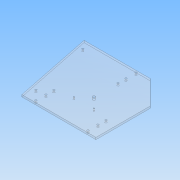
# Autodesk Inventor part: Top_Separator Backboard 2 Lanes
Saved by Autodesk Inventor 2018.1 (Build 221171000, 171)
## iProperties
Created: 2019-03-20
Part Number: Top_Separator Backboard 2 Lanes
Material: PMMA Plastic
Document SubType Name: Modeling
Designer: James
Density: 1.188 g/cm^3
Appearance: Polycarbonate - Clear
Author: James
Autodesk Inventor part; units mm, degrees
ref_plane "YZ Plane" through (0, 0, 0) normal (1, 0, 0) x (0, 1, 0)
ref_plane "XZ Plane" through (0, 0, 0) normal (0, 1, 0) x (-1, 0, 0)
ref_plane "XY Plane" through (0, 0, 0) normal (0, 0, 1) x (1, 0, 0)
sketch "Sketch1" plane through (0, 0, 0) normal (0, 0, 1) x (1, 0, 0)
  line L0 (0, 0) -> (-39.6732, 195)
  line L1 (-39.6732, 195) -> (185, 195)
  line L2 (185, 195) -> (185, 0)
  line L3 (185, 0) -> (0, 0)
  dimension "d0" = 195
  dimension "d1" = 78.5
  dimension "d2" = 185
  constraints: 8 end point, 2 perpendicular, 1 horizontal
  measures "d0" distance of L1.end L2.end
  measures "d1" angle of L3 L0
  measures "d2" distance of L2.end L0.start
extrude "Extrusion1" add sketch "Sketch1" along normal blind 5
sketch "Sketch2" plane through (0, 0, 5) normal (0, 0, 1) x (1, 0, 0)
  line L0 (0, 0) -> (185, 0) projected
  point P0 (95, 165)
  point P1 (95, 145)
  point P2 (30, 50)
  point P3 (30, 30)
  point P4 (160, 50)
  point P5 (160, 30)
  point P6 (95, 190)
  point P7 (30, 5)
  point P8 (160, 5)
  dimension "d5" = 20
  dimension "d7" = 20
  dimension "d15" = 25
  dimension "d16" = 95
  dimension "d20" = 5
  dimension "d21" = 30
  dimension "d89" = 130
  dimension "d90" = 65
  dimension "d91" = 25
  constraints: 6 vertical alignment, 3 horizontal alignment
  measures "d5" distance of point (160, 30) point (160, 50)
  measures "d7" distance of point (95, 145) point (95, 165)
  measures "d15" distance of point (95, 190) point (95, 165)
  measures "d16" vertical distance of point (160, 50) point (95, 145)
  measures "d20" distance from line of L0 point (30, 5)
  measures "d21" horizontal distance of point (30, 5) L0.start
  measures "d89" distance of point (160, 30) point (30, 30)
  measures "d90" horizontal distance of point (95, 145) point (30, 50)
  measures "d91" distance of point (160, 30) point (160, 5)
hole "Hole1" at (95, 165, 5) at (95, 145, 5) at (30, 50, 5) at (30, 30, 5) at (160, 50, 5) at (160, 30, 5) at (95, 190, 5) at (30, 5, 5) at (160, 5, 5) direction (0, 0, -1) diameter 4.5 end through all clearance for "Flat Head Machine Screw" size "M4" standard "Ansi Metric M Profile"
sketch "Sketch3" plane through (0, 0, 5) normal (0, 0, 1) x (1, 0, 0)
  circle A0 centre (30, 5) radius 2.25 projected
  circle A1 centre (160, 30) radius 2.25 projected
  circle A2 centre (30, 30) radius 2.25 projected
  circle A3 centre (95, 145) radius 2.25 projected
  circle A4 centre (95, 165) radius 2.25 projected
  circle A5 centre (30, 50) radius 2.25 projected
  circle A6 centre (160, 50) radius 2.25 projected
  line L0 (-39.6732, 195) -> (0, 0) projected
  line L1 (0, 0) -> (185, 0) projected
  line L2 (185, 0) -> (185, 195) projected
  line L3 (185, 195) -> (-39.6732, 195) projected
  point P0 (95, 85)
  dimension "d37" = 60
  constraints: 1 vertical alignment
  measures "d37" distance of A3.centre point (95, 85)
hole "Hole2" at (95, 85, 5) direction (0, 0, -1) diameter 7 end through all
sketch "Sketch4" plane through (0, 0, 5) normal (0, 0, 1) x (1, 0, 0)
  circle A0 centre (95, 85) radius 3.5 projected
  circle A1 centre (30, 5) radius 2.25 projected
  circle A2 centre (160, 30) radius 2.25 projected
  circle A3 centre (30, 30) radius 2.25 projected
  circle A4 centre (95, 145) radius 2.25 projected
  circle A5 centre (95, 165) radius 2.25 projected
  circle A6 centre (30, 50) radius 2.25 projected
  circle A7 centre (160, 50) radius 2.25 projected
  line L0 (-39.6732, 195) -> (0, 0) projected
  line L1 (0, 0) -> (185, 0) projected
  line L2 (185, 0) -> (185, 195) projected
  line L3 (185, 195) -> (-39.6732, 195) projected
  point P0 (120, 60)
  point P1 (70, 60)
  dimension "d46" = 25
  dimension "d47" = 25
  dimension "d48" = 50
  constraints: 1 horizontal alignment
  measures "d46" horizontal distance of A0.centre point (70, 60)
  measures "d47" horizontal distance of A0.centre point (70, 60)
  measures "d48" distance of point (120, 60) point (70, 60)
hole "Hole3" at (120, 60, 5) at (70, 60, 5) direction (0, 0, -1) diameter 3.4 end through all clearance for "Flat Head Machine Screw" size "M3" standard "Ansi Metric M Profile"
chamfer "Chamfer1" distance 60 angle 45 1 edges at (185, 195, 2.5)
sketch "Sketch5" plane through (0, 0, 5) normal (0, 0, 1) x (1, 0, 0)
  line L0 (-39.6732, 195) -> (0, 0) projected
  line L1 (125, 195) -> (-39.6732, 195) projected
  line L2 (0, 0) -> (185, 0) projected
  point P0 (-22.8481, 175)
  point P1 (7.0571, 28.0113)
  dimension "d64" = 12.5
  dimension "d65" = 12.5
  dimension "d66" = 150
  dimension "d67" = 20
  dimension "d68" = 28.0113
  measures "d64" distance from line of point (-22.848, 175) L0
  measures "d65" distance from line of L0 point (7.057, 28.011)
  measures "d66" distance of point (-22.848, 175) point (7.057, 28.011)
  measures "d67" distance from line of L1 point (-22.848, 175)
  measures "d68" distance from line of L2 point (7.057, 28.011)
hole "Hole4" at (-22.8481, 175, 5) at (7.0571, 28.0113, 5) direction (0, 0, -1) diameter 4.5 end through all clearance for "Flat Head Machine Screw" size "M4" standard "Ansi Metric M Profile"
sketch "Sketch6" plane through (0, 0, 5) normal (0, 0, 1) x (1, 0, 0)
  circle A0 centre (-22.8481, 175) radius 2.25 projected
  line L0 (125, 195) -> (185, 135) projected
  line L1 (125, 195) -> (-39.6732, 195) projected
  line L2 (-39.6732, 195) -> (0, 0) projected
  line L3 (0, 0) -> (185, 0) projected
  line L4 (185, 0) -> (185, 135) projected
  circle A1 centre (120, 60) radius 1.7 projected
  circle A2 centre (70, 60) radius 1.7 projected
  circle A3 centre (95, 85) radius 3.5 projected
  circle A4 centre (30, 5) radius 2.25 projected
  circle A5 centre (160, 30) radius 2.25 projected
  circle A6 centre (30, 30) radius 2.25 projected
  circle A7 centre (30, 50) radius 2.25 projected
  circle A8 centre (160, 50) radius 2.25 projected
  circle A9 centre (160, 5) radius 2.25 projected
  point P0 (30.4041, 55)
  point P1 (50, 59)
  point P2 (140, 59)
  point P3 (159.5959, 55)
  dimension "d76" = 20
  dimension "d77" = 4
  dimension "d78" = 20
  dimension "d79" = 45
  dimension "d80" = 26
  dimension "d81" = 45
  constraints: 2 horizontal alignment
  measures "d76" distance of point (50, 59) point (30.404, 55)
  measures "d77" vertical distance of point (30.404, 55) point (50, 59)
  measures "d78" distance of point (159.596, 55) point (140, 59)
  measures "d79" horizontal distance of A3.centre point (50, 59)
  measures "d80" vertical distance of A3.centre point (50, 59)
  measures "d81" horizontal distance of point (140, 59) A3.centre
hole "Hole5" [suppressed]
equation "\"d5\" = d6"
equation "\"d7\" = d5"
equation "\"d90\" = 0.5 * d89"
equation "\"d48\" = 2 * d47"
equation "\"d65\" = d64"
equation "\"d78\" = d76"
equation "\"d81\" = d79"
equation "\"d6\" = 20"
body "Solid1"
